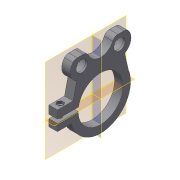
# Autodesk Inventor part: G004164_Cycl_carroZ_inferior
Saved by Autodesk Inventor 2015 SP2 (Build 190223200, 223)
## iProperties
Created: 2015-04-21
Part Number: G004164_Cycl_carroZ_inferior
Material: Genérico
Document SubType Name: Modeling
Designer: EDU
Density: 1 g/cm^3
Appearance: Valor por defecto
Author: EDU
Autodesk Inventor part; units mm, degrees
sketch "Boceto1" plane through (0, 0, 0) normal (1, 0, 0) x (0, 1, 0)
  circle A0 centre (0, 0) radius 23.75
  arc A1 (-29.376, 12.0463) -> (29.376, 12.0463) centre (0, 0) ccw
  line L0 (-29.376, 12.0463) -> (-25.5135, 29.0609)
  line L1 (29.376, 12.0463) -> (25.5135, 29.0609)
  circle A2 centre (-20, 40) radius 7.75
  circle A3 centre (20, 40) radius 7.75
  arc A4 (-12.8312, 46.4) -> (12.8312, 46.4) centre (0, 52) ccw
  line L2 (-24.8023, 50) -> (-18.3303, 50)
  arc A5 (-29.4126, 47.84) -> (-25.5135, 29.0609) centre (-20, 40) ccw
  arc A6 (25.5135, 29.0609) -> (29.4126, 47.84) centre (20, 40) ccw
  line L3 (18.3303, 50) -> (24.8023, 50)
  arc A7 (18.3303, 50) -> (12.8312, 46.4) centre (18.3303, 44) ccw
  arc A8 (-12.8312, 46.4) -> (-18.3303, 50) centre (-18.3303, 44) ccw
  arc A9 (-24.8023, 50) -> (-29.4126, 47.84) centre (-24.8023, 44) ccw
  arc A10 (29.4126, 47.84) -> (24.8023, 50) centre (24.8023, 44) ccw
  point P0 (-27.0755, 50)
  point P1 (-32.25, 40)
  point P2 (32.25, 40)
  point P3 (-27.75, 40)
  point P4 (27.75, 40)
  point P5 (-13.8564, 50)
  point P6 (13.8564, 50)
  point P7 (0, 38)
  point P8 (27.0755, 50)
  dimension "d4" = 15.5
  dimension "d5" = 15.5
  dimension "d0" = 47.5
  dimension "d1" = 63.5
  dimension "d2" = 25.58
  dimension "d7" = 4.5
  dimension "d8" = 4.5
  dimension "d25" = 51.027
  dimension "d55" = 10
  dimension "d58" = 40
  dimension "d59" = 20
  dimension "d60" = 40
  dimension "d61" = 52
  dimension "d62" = 14
  dimension "d63" = 6
  dimension "d64" = 6
  constraints: 23 point on circle, 10 horizontal alignment, 9 centre point, 8 end point, 8 tangent, 4 point on line, 3 coincident, 2 equal radius, 2 vertical alignment, 1 equal length, 1 horizontal, 5 other
  measures "d0" diameter of A0
  measures "d1" diameter of A1
  measures "d2" angle of L0 L1
  measures "d7" distance of point (32.25, 40) point (27.75, 40)
  measures "d8" distance of point (-32.25, 40) point (-27.75, 40)
  measures "d25" distance of L1.end L0.end
  measures "d55" distance from line of L2 A5.centre
  measures "d58" distance of point (-20, 40) point (20, 40)
  measures "d59" horizontal distance of point (0, 0) point (20, 40)
  measures "d60" vertical distance of point (0, 0) point (-20, 40)
  measures "d61" distance of A4.centre point (0, 0)
  measures "d62" radius of A4
  measures "d63" radius of A7
  measures "d64" radius of A9
extrude "Extrusión1" add sketch "Boceto1" along normal blind 9
sketch "Boceto2" plane through (9, 0, 0) normal (1, 0, 0) x (0, 0, -1)
  arc A0 (-12.0463, -29.376) -> (-12.0463, 29.376) centre (0, 0) ccw projected
  circle A1 centre (0, 0) radius 23.75 projected
  line L0 (7.4, -22.5677) -> (7.4, -45.7498)
  line L1 (7.4, -45.7498) -> (-0.1, -45.7498)
  line L2 (-0.1, -45.7498) -> (-0.1, -23.7498)
  circle A2 centre (0, 0) radius 23.75 projected
  line L3 (-4.1, -23.3934) -> (-4.1, -45.7498)
  line L4 (-4.1, -45.7498) -> (-12.6, -45.7498)
  line L5 (-12.6, -45.7498) -> (-12.6, -20.1321)
  line L6 (-50, -18.3303) -> (-50, -24.8023) projected
  point P0 (-50, -15.6404)
  point P1 (-50, -27.0755)
  point P2 (-29.0609, -25.5135)
  dimension "d17" = 8.5
  dimension "d18" = 7.5
  dimension "d19" = 4
  dimension "d26" = 22
  dimension "d27" = 37.4
  constraints: 12 end point, 6 point on circle, 3 vertical, 2 perpendicular, 2 point on line
  measures "d17" distance of L3.end L4.end
  measures "d18" distance of L0.end L1.end
  measures "d19" distance between parallel lines of L2 L3
  measures "d26" distance of L1.end L2.end
  measures "d27" distance between parallel lines of L5 L6
extrude "Extrusión2" add sketch "Boceto2" against normal blind 9 contours L3 L4 L5 A1 | L2 A1 L0 A0 | A0 L0 L1 L2
sketch "Boceto3" plane through (9, 0, 0) normal (1, 0, 0) x (0, 0, -1)
  circle A0 centre (-40, -20) radius 7.75 projected
  circle A1 centre (-40, 20) radius 7.75 projected
  circle A2 centre (-40, -20) radius 6
  circle A3 centre (-40, 20) radius 6
  point P0 (0, 0)
  dimension "d31" = 12
  dimension "d32" = 12
  constraints: 2 centre point, 2 coincident
  measures "d31" diameter of A2
  measures "d32" diameter of A3
extrude "Extrusión3" add sketch "Boceto3" against normal blind 2
sketch "Boceto4" plane through (9, -45.7498, -7.4) normal (0, 0, -1) x (-1, 0, 0)
  line L0 (0, 0) -> (9, 0) projected
  line L1 (9, 14.8742) -> (9, 0) projected
  point P0 (9, 45.7498)
  point P1 (4.5, 7.4371)
  point P2 (4.5, 0)
  point P3 (9, 7.4371)
  constraints: 2 midpoint, 1 horizontal alignment, 1 vertical alignment
hole "Agujero1" at (4.5, -38.3127, -7.4) direction (0, 0, 1) diameter 3.75 end through all
sketch "Boceto5" plane through (9, -45.7498, 12.6) normal (0, 0, 1) x (1, 0, 0)
  circle A0 centre (-4.5, 7.4371) radius 1.875 projected
  line L0 (-6.2999, 10.5546) -> (-2.7001, 10.5546)
  line L1 (-2.7001, 10.5546) -> (-0.9002, 7.4371)
  line L2 (-0.9002, 7.4371) -> (-2.7001, 4.3196)
  line L3 (-2.7001, 4.3196) -> (-6.2999, 4.3196)
  line L4 (-6.2999, 4.3196) -> (-8.0998, 7.4371)
  line L5 (-8.0998, 7.4371) -> (-6.2999, 10.5546)
  point P0 (-9, 45.7498)
  dimension "d44" = 6.235
  constraints: 12 end point, 1 coincident, 1 horizontal, 13 other
  measures "d44" distance between parallel lines of L4 L1
extrude "Extrusión4" cut sketch "Boceto5" against normal blind 2.8
sketch "Boceto6" plane through (0, 0, 0) normal (-1, 0, 0) x (0, 0, 1)
  line L0 (0.1, -45.7498) -> (0.1, -31.7498) projected
  line L1 (4.1, -31.4842) -> (4.1, -45.7498) projected
  line L2 (0.1, -31.7498) -> (4.1, -31.7498)
  line L3 (4.1, -31.7498) -> (4.1, -21.7498)
  line L4 (4.1, -21.7498) -> (0.1, -21.7498)
  line L5 (0.1, -21.7498) -> (0.1, -31.7498)
  point P0 (0, 0)
  dimension "d50" = 10
  constraints: 8 end point, 2 parallel, 1 horizontal, 1 perpendicular, 1 vertical alignment
  measures "d50" distance of L2.end L3.end
extrude "Extrusión5" cut sketch "Boceto6" against normal through all
equation "\"d5\" = d4"
